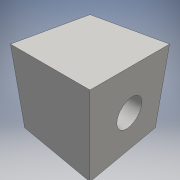
# Autodesk Inventor part: holetest
Saved by Autodesk Inventor 2016 (Build 200138000, 138)
## iProperties
Created: 2015-11-18
Part Number: holetest
Material: Generic
Document SubType Name: Modeling
Designer: hesaon
Density: 1 g/cm^3
Appearance: Default
Author: hesaon
Autodesk Inventor part; units mm, degrees
ref_plane "YZ Plane" through (0, 0, 0) normal (1, 0, 0) x (0, 1, 0)
ref_plane "XZ Plane" through (0, 0, 0) normal (0, 1, 0) x (-1, 0, 0)
ref_plane "XY Plane" through (0, 0, 0) normal (0, 0, 1) x (1, 0, 0)
sketch "Sketch1" plane through (0, 0, 0) normal (0, 0, 1) x (1, 0, 0)
  line L0 (0, 0) -> (20, 0)
  line L1 (20, 0) -> (20, 20)
  line L2 (20, 20) -> (0, 20)
  line L3 (0, 20) -> (0, 0)
  line L4 (0, 20) -> (10, 20)
  dimension "d0" = 20
  dimension "d1" = 20
  constraints: 10 end point, 2 parallel, 1 horizontal, 1 midpoint, 1 perpendicular
  measures "d0" distance of L2.end L1.end
  measures "d1" distance of L1.end L0.end
extrude "Extrusion1" add sketch "Sketch1" along normal blind 20
sketch "Sketch2" plane through (20, 0, 0) normal (1, 0, 0) x (0, 0, -1)
  circle A0 centre (-10, 10) radius 3.5
  line L0 (0, 20) -> (-20, 20) projected
  line L1 (-20, 0) -> (-20, 20) projected
  point P0 (0, 0)
  dimension "d4" = 7
  dimension "d5" = 10
  dimension "d6" = 10
  constraints: 1 centre point
  measures "d4" diameter of A0
  measures "d5" distance from line of L0 A0.centre
  measures "d6" distance from line of L1 A0.centre
extrude "Extrusion2" cut sketch "Sketch2" against normal blind 10
sketch "Sketch3" plane through (0, 0, 0) normal (-1, 0, 0) x (0, 0, 1)
  circle A0 centre (10, 10) radius 2
  line L0 (0, 0) -> (20, 0) projected
  line L1 (20, 20) -> (20, 0) projected
  dimension "d9" = 4
  dimension "d10" = 10
  dimension "d11" = 10
  constraints: 1 centre point
  measures "d9" diameter of A0
  measures "d10" distance from line of L0 A0.centre
  measures "d11" distance from line of L1 A0.centre
extrude "Extrusion3" cut sketch "Sketch3" against normal blind 10
body "Solid1"
